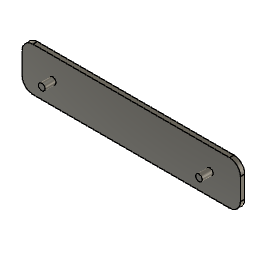
hook v3 (Autodesk Fusion 360 design; units mm, degrees)
Autodesk Fusion 360 part; units mm, degrees
sketch "Sketch1" plane through (0, 0, 0) normal (0, 1, 0) x (1, 0, 0)
  line L0 (0, -20) -> (100, -20)
  line L1 (100, -20) -> (100, 0)
  line L2 (100, 0) -> (0, 0)
  line L3 (0, 0) -> (0, -20)
  dimension "d1" = 100
  constraint horizontal L0
  constraint vertical L1
  constraint horizontal L2
  constraint vertical L3
  measures "d1" distance of L0.start L0.end
extrude "Extrude1" add sketch "Sketch1" along normal blind 2
sketch "Sketch2" plane through (0, 0, 0) normal (0, 1, 0) x (1, 0, 0)
  circle A0 centre (14, -10) radius 1.5
  dimension "d4" = 3
  measures "d4" diameter of A0
extrude "Extrude2" add sketch "Sketch2" against normal blind 5
sketch "Sketch3" plane through (0, 0, 0) normal (0, 1, 0) x (1, 0, 0)
  circle A0 centre (86, -10) radius 1.5
  dimension "d7" = 3
  measures "d7" diameter of A0
extrude "Extrude3" add sketch "Sketch3" against normal blind 5
fillet "Fillet1" radius 5 1 edges at (0, 1, 20)
fillet "Fillet2" radius 5 1 edges at (100, 1, 20)
fillet "Fillet3" radius 5 1 edges at (100, 1, 0)
fillet "Fillet4" radius 5 1 edges at (0, 1, 0)
